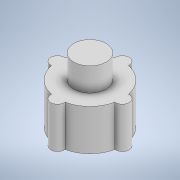
# Autodesk Inventor part: Acople Resorte-Marcador
Saved by Autodesk Inventor 2022 (Build 260153000, 153)
## iProperties
Created: 2022-08-23
Part Number: Acople Resorte-Marcador
Material: Generic
Document SubType Name: Modeling
Designer: David
Density: 1 g/cm^3
Appearance: Default
Author: David
Autodesk Inventor part; units mm, degrees
ref_plane "YZ Plane" through (0, 0, 0) normal (1, 0, 0) x (0, 1, 0)
ref_plane "XZ Plane" through (0, 0, 0) normal (0, 1, 0) x (-1, 0, 0)
ref_plane "XY Plane" through (0, 0, 0) normal (0, 0, 1) x (1, 0, 0)
sketch "Sketch1" plane through (0, 0, 0) normal (0, 1, 0) x (-1, 0, 0)
  circle A0 centre (0, 0) radius 9.5
  dimension "d0" = 19
  constraints: 1 centre point, 1 coincident
  measures "d0" diameter of A0
extrude "Extrusion1" add sketch "Sketch1" along normal blind 12
sketch "Sketch2" plane through (0, 12, 0) normal (0, 1, 0) x (1, 0, 0)
  circle A0 centre (0, 0) radius 4.7244
  dimension "d9" = 9.4488
  constraints: 1 centre point, 1 coincident
  measures "d9" diameter of A0
extrude "Extrusion2" add sketch "Sketch2" along normal blind 6.9088
sketch "Sketch3" plane through (0, 0, 0) normal (0, -1, 0) x (1, 0, 0)
  circle A0 centre (0, 0) radius 4.48
  circle A1 centre (0, 0) radius 6
  dimension "d5" = 12
  dimension "d6" = 1.52
  constraints: 2 centre point, 2 coincident
  measures "d5" diameter of A1
  measures "d6" radial gap between concentric circles of A1 A0
extrude "Extrusion3" cut sketch "Sketch3" against normal blind 3
sketch "Sketch4" plane through (0, 12, 0) normal (0, 1, 0) x (1, 0, 0)
  circle A0 centre (0, 0) radius 9.5 projected
  circle A1 centre (-9.5, 0) radius 2
  line L0 (-15.7, 0) -> (13.7, 0) projected
  point P0 (-9.2895, 1.9889)
  point P1 (-9.2895, -1.9889)
  dimension "d10" = 4
  constraints: 1 centre point, 1 point on line, 2 other
  measures "d10" diameter of A1
extrude "Extrusion4" add sketch "Sketch4" against normal up to surface (12 mm away) contours A0 L0 A1 | A1 L0 A0 picked at (-10.0838, 0.5297) picked at (-10.0838, -0.5297)
pattern_circular "Circular Pattern1" count 4 over 360 about axis through (0, 0, 0) along (0, 1, 0) of "Extrusion4"
body "Solid1"
